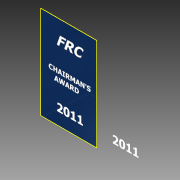
# Autodesk Inventor part: Chairmans Award Banner
Saved by Autodesk Inventor 2014 (Build 180170000, 170)
## iProperties
Created: 2015-04-18
Part Number: Chairmans Award Banner
Material: Generic
Document SubType Name: Modeling
Designer: Gus
Density: 1 g/cm^3
Appearance: Default
Author: Gus
Autodesk Inventor part; units mm, degrees
ref_plane "YZ Plane" through (0, 0, 0) normal (1, 0, 0) x (0, 1, 0)
ref_plane "XZ Plane" through (0, 0, 0) normal (0, 1, 0) x (-1, 0, 0)
ref_plane "XY Plane" through (0, 0, 0) normal (0, 0, 1) x (1, 0, 0)
sketch "Sketch1" plane through (0, 0, 0) normal (0, 0, 1) x (1, 0, 0)
  line L0 (0, 0) -> (914.4, 0)
  line L1 (914.4, 0) -> (914.4, 1524)
  line L2 (914.4, 1524) -> (0, 1524)
  line L3 (0, 1524) -> (0, 0)
  dimension "d0" = 914.4
  dimension "d1" = 1524
  constraints: 8 end point, 2 parallel, 1 horizontal, 1 perpendicular
  measures "d0" distance of L2.end L1.end
  measures "d1" distance of L1.end L0.end
extrude "Extrusion1" add sketch "Sketch1" along normal blind 5.08
sketch "Sketch2" plane through (0, 0, 5.08) normal (0, 0, 1) x (1, 0, 0)
  line L0 (0, 0) -> (914.4, 0) projected
  line L1 (914.4, 0) -> (914.4, 1524) projected
  line L2 (914.4, 1524) -> (0, 1524) projected
  line L3 (0, 1524) -> (0, 0) projected
  line L4 (131.852, 815.5661) -> (1123.0489, 815.5661) construction
  line L5 (1123.0489, 815.5661) -> (1123.0489, 473.8035) construction
  line L6 (1123.0489, 473.8035) -> (131.852, 473.8035) construction
  line L7 (131.852, 473.8035) -> (131.852, 815.5661) construction
  line L8 (250.4439, 1292.9292) -> (615.6358, 1292.9292) construction
  line L9 (615.6358, 1292.9292) -> (615.6358, 1135.0952) construction
  line L10 (615.6358, 1135.0952) -> (250.4439, 1135.0952) construction
  line L11 (250.4439, 1135.0952) -> (250.4439, 1292.9292) construction
  constraints: 4 other
sketch "Sketch3" plane through (0, 0, 5.08) normal (0, 0, 1) x (1, 0, 0)
  line L0 (0, 0) -> (914.4, 0) projected
  line L1 (914.4, 0) -> (914.4, 1524) projected
  line L2 (914.4, 1524) -> (0, 1524) projected
  line L3 (0, 1524) -> (0, 0) projected
  line L4 (258.5063, 325.7377) -> (639.7121, 325.7377) construction
  line L5 (639.7121, 325.7377) -> (639.7121, 193.386) construction
  line L6 (639.7121, 193.386) -> (258.5063, 193.386) construction
  line L7 (258.5063, 193.386) -> (258.5063, 325.7377) construction
  line L8 (1169.6792, 324.1112) -> (1550.885, 324.1112) construction
  line L9 (1550.885, 324.1112) -> (1550.885, 191.7595) construction
  line L10 (1550.885, 191.7595) -> (1169.6792, 191.7595) construction
  line L11 (1169.6792, 191.7595) -> (1169.6792, 324.1112) construction
  constraints: 4 other
body "Solid1"
